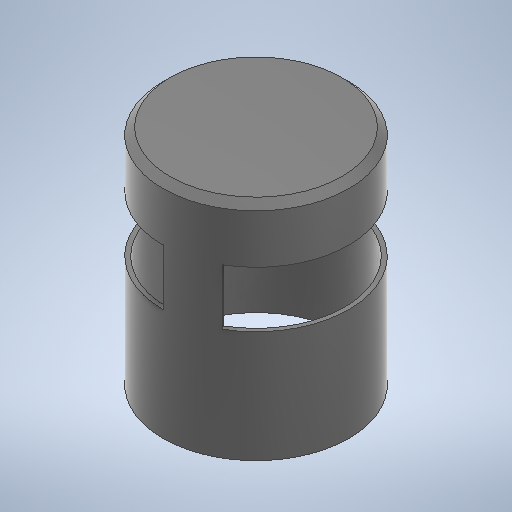
# Autodesk Inventor part: siren_new
Saved by Autodesk Inventor 2026.2 (Build 302298010, 298A)
## iProperties
Created: 2026-05-28
Part Number: siren_new
Material: ABS Plastic
Document SubType Name: Modeling
Designer: chris
Density: 1.06 g/cm^3
Appearance: Smooth - White
Author: chris
Autodesk Inventor part; units mm, degrees
ref_plane "YZ Plane" through (0, 0, 0) normal (1, 0, 0) x (0, 1, 0)
sketch "Sketch1" plane through (0, 0, 0) normal (0, 1, 0) x (-1, 0, 0)
  circle A0 centre (0, 0) radius 63.5
  circle A1 centre (0, 0) radius 66.5
  dimension "d0" = 127
  dimension "d1" = 133
  constraints: 2 centre point, 2 coincident
  measures "d0" diameter of A0
  measures "d1" diameter of A1
extrude "Extrusion1" add sketch "Sketch1" along normal blind 160
ref_plane "Work Plane1" through (0, 160, 0) normal (0, 1, 0) x (-1, 0, 0)
sketch "Sketch2" plane through (0, 160, 0) normal (0, 1, 0) x (-1, 0, 0)
  circle A0 centre (0, 0) radius 63.5
  dimension "d5" = 127
  constraints: 1 centre point, 1 coincident
  measures "d5" diameter of A0
extrude "Extrusion2" add sketch "Sketch2" against normal blind 3
chamfer "Chamfer1" distance 5 angle 45 1 edges at (66.5, 160, 0)
chamfer "Chamfer2" distance 5 angle 45 1 edges at (63.5, 157, 0)
ref_plane "Work Plane2" through (0, 80, 0) normal (0, 1, 0) x (-1, 0, 0)
sketch "Sketch3" plane through (0, 80, 0) normal (0, 1, 0) x (-1, 0, 0)
  circle A0 centre (0, 0) radius 63.5
  circle A1 centre (0, 0) radius 66.5
  line L0 (0, 0) -> (0, -66.5)
  line L1 (0, 0) -> (33.25, -57.5907)
  line L2 (0, 0) -> (66.5, 0) construction
  line L3 (0, 0) -> (0, 66.5)
  line L4 (0, 0) -> (-33.25, 57.5907)
  point P0 (0, 63.5)
  point P1 (31.75, -54.9926)
  point P2 (-31.75, 54.9926)
  point P3 (0, -63.5)
  dimension "d15" = 127
  dimension "d16" = 133
  dimension "d17" = 60
  constraints: 10 end point, 4 point on circle, 2 centre point, 2 coincident, 1 equal length, 1 horizontal, 1 perpendicular, 1 vertical
  measures "d15" diameter of A0
  measures "d16" diameter of A1
  measures "d17" angle of L1 L2
extrude "Extrusion3" cut sketch "Sketch3" along normal blind 40 contours A0 L3 A1 L1 | A0 L0 A1 L4
body "Solid1"
